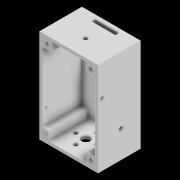
# Autodesk Inventor part: Parte de abajo contenedor
Saved by Autodesk Inventor 2020 (Build 240168000, 168)
## iProperties
Created: 2021-12-09
Part Number: Parte de abajo contenedor
Material: Generic
Document SubType Name: Modeling
Designer: juan
Density: 1 g/cm^3
Appearance: Default
Author: juan
Autodesk Inventor part; units mm, degrees
ref_plane "YZ Plane" through (0, 0, 0) normal (1, 0, 0) x (0, 1, 0)
ref_plane "XZ Plane" through (0, 0, 0) normal (0, 1, 0) x (-1, 0, 0)
ref_plane "XY Plane" through (0, 0, 0) normal (0, 0, 1) x (1, 0, 0)
sketch "Sketch1" plane through (0, 0, 0) normal (0, 0, 1) x (1, 0, 0)
  line L0 (0, 0) -> (49.5, 0)
  line L1 (49.5, 0) -> (49.5, 79)
  line L2 (49.5, 79) -> (0, 79)
  line L3 (0, 79) -> (0, 0)
  dimension "d0" = 49.5
  dimension "d1" = 79
  constraints: 8 end point, 2 parallel, 1 horizontal, 1 perpendicular
  measures "d0" distance of L2.end L1.end
  measures "d1" distance of L2.end L0.start
extrude "Extrusion1" add sketch "Sketch1" along normal blind 35.867
sketch "Sketch2" plane through (0, 0, 35.867) normal (0, 0, 1) x (1, 0, 0)
  line L0 (0, 79) -> (0, 0) construction
  line L1 (49.5, 79) -> (0, 79) construction
  line L2 (49.5, 0) -> (49.5, 79) construction
  line L3 (0, 0) -> (49.5, 0) construction
  line L4 (2.5, 2.5) -> (47, 2.5)
  line L5 (47, 2.5) -> (47, 76.5)
  line L6 (47, 76.5) -> (2.5, 76.5)
  line L7 (2.5, 76.5) -> (2.5, 2.5)
  dimension "d4" = 2.5
  dimension "d5" = 2.5
  dimension "d6" = 2.5
  dimension "d7" = 2.5
  constraints: 8 end point, 2 parallel, 1 horizontal, 1 perpendicular
  measures "d4" distance between parallel lines of L1 L6
  measures "d5" distance between parallel lines of L0 L7
  measures "d6" distance between parallel lines of L4 L3
  measures "d7" distance between parallel lines of L2 L5
extrude "Extrusion2" cut sketch "Sketch2" against normal blind 32.367
sketch "Sketch3" plane through (0, 0, 0) normal (0, -1, 0) x (1, 0, 0)
  line L0 (0, 0) -> (49.5, 0) construction
  line L1 (49.5, 0) -> (49.5, 35.867) construction
  line L2 (0, 35.867) -> (49.5, 35.867) construction
  line L3 (0, 0) -> (0, 35.867) construction
  point P0 (21.75, 18.5)
  point P1 (24.75, 35.867)
  dimension "d12" = 17.367
  dimension "d31" = 21.75
  constraints: 1 midpoint
  measures "d12" distance from line of L2 point (21.75, 18.5)
  measures "d31" distance from line of L3 point (21.75, 18.5)
hole "Hole1" at (21.75, 0, 18.5) direction (0, 1, 0) diameter 7.1 depth 2.5 tip angle 118
sketch "Sketch4" plane through (0, 0, 0) normal (0, -1, 0) x (1, 0, 0)
  circle A0 centre (21.75, 18.5) radius 3.55 construction
  line L0 (0, 0) -> (49.5, 0) construction
  line L1 (49.5, 0) -> (49.5, 35.867) construction
  line L2 (0, 35.867) -> (49.5, 35.867) construction
  line L3 (0, 0) -> (0, 35.867) construction
  point P0 (21.75, 27)
  dimension "d20" = 8.5
  measures "d20" distance of point (21.75, 27) A0.centre
hole "Hole2" at (21.75, 0, 27) direction (0, 1, 0) diameter 3.3 depth 2.5 tip angle 118
pattern_circular "Circular Pattern1" count 4 over 360 about axis through (21.75, 99.8884, 18.5) along (0, -1, 0) of "Hole2"
sketch "Sketch5" plane through (0, 0, 0) normal (-1, 0, 0) x (0, 0, 1)
  line L0 (35.867, 79) -> (35.867, 0) projected
  line L1 (0, 0) -> (35.867, 0) projected
  point P0 (32.881, 22.9529)
  point P1 (10.021, 53.4329)
  dimension "d32" = 2.986
  dimension "d33" = 30.48
  dimension "d34" = 22.86
  dimension "d35" = 22.9529
  measures "d32" distance from line of L0 point (32.881, 22.953)
  measures "d33" vertical distance of point (32.881, 22.953) point (10.021, 53.433)
  measures "d34" horizontal distance of point (10.021, 53.433) point (32.881, 22.953)
  measures "d35" distance from line of L1 point (32.881, 22.953)
hole "Hole3" at (0, 22.9529, 32.881) at (0, 53.4329, 10.021) direction (1, 0, 0) diameter 2.184 depth 2.5 tip angle 118
fillet "Fillet3" radius 2 3 edges at (24.75, 2.5, 3.5) (47, 2.5, 19.6835) (2.5, 2.5, 19.6835)
sketch "Sketch6" plane through (49.5, 0, 0) normal (1, 0, 0) x (0, 0, -1)
  line L0 (-35.867, 0) -> (-35.867, 79) projected
  line L1 (0, 79) -> (-35.867, 79) projected
  point P0 (0, 0)
  point P1 (-16.667, 23)
  point P2 (-32.667, 53)
  dimension "d44" = 30
  dimension "d47" = 26
  dimension "d55" = 3.2
  dimension "d56" = 16
  measures "d44" vertical distance of point (-32.667, 53) point (-16.667, 23)
  measures "d47" distance from line of L1 point (-32.667, 53)
  measures "d55" distance from line of L0 point (-32.667, 53)
  measures "d56" horizontal distance of point (-32.667, 53) point (-16.667, 23)
hole "Hole4" at (49.5, 23, 16.667) at (49.5, 53, 32.667) direction (-1, 0, 0) diameter 3 depth 2.5 tip angle 118
sketch "Sketch7" plane through (0, 0, 35.867) normal (0, 0, 1) x (1, 0, 0)
  line L0 (49.5, 0) -> (39.5, 0)
  line L1 (39.5, 0) -> (39.5, 10)
  line L2 (39.5, 10) -> (49.5, 10)
  line L3 (49.5, 10) -> (49.5, 0)
  line L4 (0, 0) -> (8, 0)
  line L5 (8, 0) -> (8, 10)
  line L6 (8, 10) -> (0, 10)
  line L7 (0, 10) -> (0, 0)
  line L8 (0, 79) -> (10, 79)
  line L9 (10, 79) -> (10, 69)
  line L10 (10, 69) -> (0, 69)
  line L11 (0, 69) -> (0, 79)
  line L12 (49.5, 79) -> (39.5, 79)
  line L13 (39.5, 79) -> (39.5, 69)
  line L14 (39.5, 69) -> (49.5, 69)
  line L15 (49.5, 69) -> (49.5, 79)
  line L16 (49.5, 79) -> (0, 79) projected
  line L17 (49.5, 0) -> (49.5, 79) projected
  point P0 (4, 0)
  point P1 (44.5, 0)
  point P2 (5, 79)
  point P3 (44.5, 79)
  point P4 (49.5, 74)
  point P5 (49.5, 5)
  point P6 (0, 74)
  point P7 (0, 5)
  point P8 (24.75, 79)
  point P9 (49.5, 39.5)
  dimension "d57" = 10
  dimension "d58" = 8
  dimension "d59" = 10
  dimension "d60" = 10
  dimension "d61" = 10
  dimension "d62" = 10
  dimension "d63" = 10
  dimension "d64" = 10
  constraints: 32 end point, 10 midpoint, 8 parallel, 4 horizontal, 4 perpendicular, 3 horizontal alignment, 3 point on line, 3 vertical alignment
  measures "d57" distance of L1.end L2.end
  measures "d58" distance of L6.end L5.end
  measures "d59" distance of L9.end L10.end
  measures "d60" distance of L14.end L13.end
  measures "d61" distance of L0.end L1.end
  measures "d62" distance of L4.end L5.end
  measures "d63" distance of L10.end L8.start
  measures "d64" distance of L14.end L12.start
extrude "Extrusion3" add sketch "Sketch7" against normal up to surface (32.367 mm away)
sketch "Sketch8" plane through (0, 0, 35.867) normal (0, 0, 1) x (1, 0, 0)
  line L0 (39.5, 2.5) -> (8, 2.5) construction
  line L1 (8, 2.5) -> (8, 10) construction
  line L2 (8, 10) -> (2.5, 10) construction
  line L3 (2.5, 10) -> (2.5, 69) construction
  line L4 (2.5, 69) -> (10, 69) construction
  line L5 (10, 69) -> (10, 76.5) construction
  line L6 (10, 76.5) -> (39.5, 76.5) construction
  line L7 (39.5, 76.5) -> (39.5, 69) construction
  line L8 (39.5, 69) -> (47, 69) construction
  line L9 (47, 69) -> (47, 10) construction
  line L10 (47, 10) -> (39.5, 10) construction
  line L11 (39.5, 10) -> (39.5, 2.5) construction
  line L12 (49.5, 79) -> (0, 79) construction
  line L13 (0, 79) -> (0, 0) construction
  line L14 (0, 0) -> (49.5, 0) construction
  line L15 (49.5, 0) -> (49.5, 79) construction
  point P0 (5.25, 6.25)
  point P1 (43.25, 6.25)
  point P2 (43.25, 72.75)
  point P3 (6.25, 72.75)
  point P4 (5.25, 10)
  point P5 (8, 6.25)
  point P6 (39.5, 6.25)
  point P7 (39.5, 72.75)
  point P8 (10, 72.75)
  point P9 (6.25, 69)
  point P10 (43.25, 69)
  point P11 (43.25, 10)
  constraints: 8 midpoint, 4 horizontal alignment, 4 vertical alignment
hole "Hole5" at (5.25, 6.25, 35.867) at (43.25, 6.25, 35.867) at (43.25, 72.75, 35.867) at (6.25, 72.75, 35.867) direction (0, 0, -1) diameter 3.3 end through all
sketch "Sketch9" plane through (0, 79, 0) normal (0, 1, 0) x (1, 0, 0)
  line L0 (49.5, -35.867) -> (0, -35.867) projected
  point P0 (0, 0)
  point P1 (24.75, -21.639)
  point P2 (24.75, -35.867)
  dimension "d75" = 14.228
  constraints: 1 midpoint, 1 vertical alignment
  measures "d75" distance from line of L0 point (24.75, -21.639)
hole "Hole6" at (24.75, 79, 21.639) direction (0, -1, 0) diameter 3.3 depth 2.5 tip angle 118
sketch "Sketch10" plane through (10, 76.5, 35.867) normal (0, -1, 0) x (1, 0, 0)
  line L0 (0, -32.367) -> (29.5, -32.367) construction
  circle A0 centre (14.75, -14.228) radius 1.65 construction
  line L1 (0, 0) -> (0, -32.367) construction
  line L2 (0, -32.367) -> (29.5, -32.367) construction
  line L3 (29.5, -32.367) -> (29.5, 0) construction
  line L4 (0, 0) -> (29.5, 0) construction
  line L5 (24.75, -32.367) -> (4.75, -32.367)
  line L6 (4.75, -32.367) -> (4.75, -29.367)
  line L7 (4.75, -29.367) -> (24.75, -29.367)
  line L8 (24.75, -29.367) -> (24.75, -32.367)
  point P0 (-10, -35.867)
  point P1 (14.75, -29.367)
  point P2 (14.75, 0)
  dimension "d83" = 20
  dimension "d84" = 3
  constraints: 8 end point, 2 midpoint, 2 parallel, 1 horizontal, 1 perpendicular, 1 point on line, 1 vertical alignment
  measures "d83" distance of L6.end L7.end
  measures "d84" distance of L7.end L5.start
extrude "Extrusion4" cut sketch "Sketch10" against normal through all
body "Solid1"
